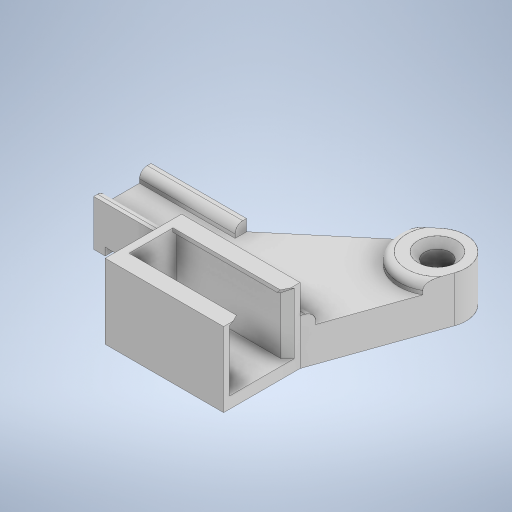
# Autodesk Inventor part: Strain Relief
Saved by Autodesk Inventor 2023.1 (Build 271208000, 208)
## iProperties
Created: 2022-11-07
Part Number: Strain Relief
Material: Generic
Document SubType Name: Modeling
Designer: nicol
Density: 1 g/cm^3
Appearance: Default
Author: nicol
Autodesk Inventor part; units mm, degrees
ref_plane "YZ Plane" through (0, 0, 0) normal (1, 0, 0) x (0, 1, 0)
ref_plane "XZ Plane" through (0, 0, 0) normal (0, 1, 0) x (-1, 0, 0)
ref_plane "XY Plane" through (0, 0, 0) normal (0, 0, 1) x (1, 0, 0)
sketch "Sketch1" plane through (0, 0, 0) normal (0, 1, 0) x (-1, 0, 0)
  circle A0 centre (-32.475, -32.475) radius 3.3
  circle A1 centre (-32.475, -32.475) radius 7.5
  line L0 (25, 0) -> (0, 0)
  line L1 (0, 0) -> (0, -15)
  line L2 (0, -15) -> (25, -15)
  line L3 (25, -15) -> (25, 0)
  line L4 (0, 20) -> (-29, 20)
  line L5 (-29, 20) -> (-29, 0)
  line L6 (-29, 0) -> (0, 0)
  line L7 (0, 0) -> (0, 20)
  line L8 (0, 0) -> (-36.8411, -26.3768)
  line L9 (0, -15) -> (-27.6522, -38.2187)
  line L10 (-29, 0) -> (-39.5499, -29.9858)
  line L11 (0, 0) -> (-55.6524, 0) construction
  line L12 (-55.6524, 0) -> (-55.6524, -63.0935) construction
  line L13 (-55.6524, -63.0935) -> (0, -63.0935) construction
  line L14 (0, -63.0935) -> (0, 0) construction
  dimension "d0" = 6.6
  dimension "d1" = 32.475
  dimension "d2" = 32.475
  dimension "d3" = 15
  dimension "d4" = 25
  dimension "d6" = 15
  dimension "d7" = 29
  dimension "d8" = 20
  constraints: 30 end point, 6 parallel, 3 horizontal, 3 perpendicular, 3 point on circle, 3 tangent, 2 centre point, 2 coincident, 2 collinear
  measures "d0" diameter of A0
  measures "d1" distance from line of A0.centre L14
  measures "d2" distance from line of L11 A0.centre
  measures "d3" distance of L2.end L0.start
  measures "d4" distance of L1.end L2.end
  measures "d6" diameter of A1
  measures "d7" distance of L4.start L4.end
  measures "d8" distance of L6.end L4.start
extrude "Extrusion1" add sketch "Sketch1" along normal blind 12
sketch "Sketch2" plane through (0, 12, 0) normal (0, 1, 0) x (1, 0, 0)
  circle A0 centre (32.475, 32.475) radius 3.3 projected
  circle A1 centre (32.475, 32.475) radius 10
  line L0 (-25, 15) -> (-25, 0) projected
  line L1 (-25, 0) -> (0, 0) projected
  line L2 (0, 0) -> (0, -20) projected
  line L3 (0, -20) -> (29, -20) projected
  line L4 (29, -20) -> (29, 0) projected
  line L5 (29, 0) -> (39.5499, 29.9858) projected
  arc A2 (39.5499, 29.9858) -> (27.6522, 38.2187) centre (32.475, 32.475) ccw projected
  line L6 (27.6522, 38.2187) -> (0, 15) projected
  line L7 (0, 15) -> (-25, 15) projected
  circle A3 centre (32.475, 32.475) radius 3.3 projected
  line L8 (-25, 15) -> (-25, 0) projected
  line L9 (-25, 12) -> (0, 12)
  line L10 (0, 12) -> (0, 3)
  line L11 (0, 3) -> (-25, 3)
  line L12 (-25, 3) -> (-25, 12)
  line L13 (27.6522, 38.2187) -> (0, 15) projected
  line L14 (0, 15) -> (0, 0)
  line L15 (29, 0) -> (39.5499, 29.9858) projected
  line L16 (0, 0) -> (30.0555, 0)
  line L17 (30.0555, 0) -> (30.0555, 3)
  line L18 (30.0555, 3) -> (0, 3)
  line L19 (0, 3) -> (0, 0)
  point P0 (37.3547, 23.7464)
  point P1 (22.5867, 33.9654)
  point P2 (-25, 7.5)
  point P3 (-25, 3)
  point P4 (29, 0)
  point P5 (29, 0)
  dimension "d11" = 20
  dimension "d14" = 9
  constraints: 18 end point, 4 parallel, 3 point on line, 2 horizontal, 2 midpoint, 2 perpendicular, 1 centre point, 1 coincident, 1 collinear, 1 vertical
  measures "d11" diameter of A1
  measures "d14" distance of L9.end L10.end
extrude "Extrusion2" cut sketch "Sketch2" against normal blind 3 contours A1 L5 L18 L10 L14 L6 | L17 L16 L5 | L10 L11 L0 L9
extrude "Extrusion7" cut sketch "Sketch2" against normal blind 9 contours L4 L3 L2 L16
sketch "Sketch3" plane through (0, 3, 0) normal (0, 1, 0) x (1, 0, 0)
  line L0 (0, -16.75) -> (29, -16.75)
  line L1 (29, -16.75) -> (29, -3.25)
  line L2 (29, -3.25) -> (0, -3.25)
  line L3 (0, -3.25) -> (0, -16.75)
  line L4 (37.3547, 23.7464) -> (30.0555, 3) projected
  arc A0 (22.5867, 33.9654) -> (37.3547, 23.7464) centre (32.475, 32.475) ccw projected
  line L5 (0, 15) -> (22.5867, 33.9654) projected
  line L6 (0, 12) -> (0, 15) projected
  line L7 (-25, 12) -> (0, 12) projected
  line L8 (-25, 3) -> (-25, 12) projected
  line L9 (30.0555, 3) -> (-25, 3) projected
  line L10 (0, 0) -> (29, 0)
  line L11 (29, 0) -> (29, -20) projected
  line L12 (0, 0) -> (29, 0) projected
  line L13 (0, -20) -> (0, 0) projected
  line L14 (29, -20) -> (0, -20) projected
  point P0 (29, -10)
  point P1 (0, -10)
  point P2 (0, -3.25)
  dimension "d15" = 13.5
  constraints: 10 end point, 3 midpoint, 2 horizontal, 2 parallel, 1 perpendicular
  measures "d15" distance of L1.end L0.end
extrude "Extrusion3" add sketch "Sketch3" along normal blind 16.5 contours L0 L11 L14 L13 | L13 L10 L11 L2
sketch "Sketch4" plane through (29, 0, 20) normal (1, 0, 0) x (0, 0, -1)
  line L0 (3.25, 19.5) -> (4.25, 19.5)
  line L1 (16.75, 19.5) -> (15.75, 19.5)
  line L2 (0, 0) -> (0, 19.5) projected
  line L3 (0, 0) -> (20, 0) projected
  line L4 (20, 0) -> (20, 12) projected
  line L5 (4.25, 19.5) -> (4.25, 18.5)
  line L6 (4.25, 18.5) -> (3.25, 17.9226)
  line L7 (15.75, 19.5) -> (15.75, 18.5)
  line L8 (15.75, 18.5) -> (16.75, 17.9226)
  line L9 (16.75, 3) -> (3.25, 3) projected
  line L10 (3.25, 3) -> (3.25, 19.5) projected
  line L11 (0, 19.5) -> (3.25, 19.5) projected
  line L12 (20, 12) -> (20, 19.5) projected
  line L13 (16.75, 19.5) -> (20, 19.5) projected
  line L14 (16.75, 3) -> (16.75, 19.5) projected
  line L15 (16.75, 3) -> (16.75, 19.5) projected
  point P0 (3.25, 23.5)
  point P1 (16.75, 23.5)
  dimension "d18" = 1
  dimension "d20" = 1
  dimension "d27" = 1
  dimension "d28" = 120
  dimension "d29" = 1
  dimension "d30" = 120
  constraints: 12 end point, 2 horizontal, 2 vertical, 1 point on line
  measures "d18" distance of L1.start L1.end
  measures "d20" distance of L0.start L0.end
  measures "d27" distance of L1.end L7.end
  measures "d28" angle of L7 L8
  measures "d29" distance of L0.end L5.end
  measures "d30" angle of L6 L5
extrude "Extrusion4" add sketch "Sketch4" against normal up to surface (29 mm away) contours L0 L5 L6 L10 | L8 L7 L1 L14
sketch "Sketch5" plane through (0, 0, 0) normal (-1, 0, 0) x (0, 0, 1)
  line L0 (0, 0) -> (20, 0) projected
  line L1 (0, 19.5) -> (4.25, 19.5) projected
  line L2 (3.25, 19.5) -> (16.75, 19.5)
  line L3 (0, 0) -> (0, 12) projected
  line L4 (16.75, 3) -> (3.25, 3) projected
  line L5 (3.25, 3) -> (3.25, 17.9226) projected
  line L6 (0, 12) -> (0, 19.5) projected
  line L7 (20, 0) -> (20, 19.5) projected
  line L8 (15.75, 19.5) -> (20, 19.5) projected
  line L9 (16.75, 3) -> (16.75, 17.9226) projected
  line L10 (4.25, 18.5) -> (3.25, 17.9226) projected
  line L11 (4.25, 19.5) -> (4.25, 18.5) projected
  line L12 (15.75, 18.5) -> (15.75, 19.5) projected
  line L13 (16.75, 17.9226) -> (15.75, 18.5) projected
  constraints: 2 end point
extrude "Extrusion5" add sketch "Sketch5" along normal blind 2
sketch "Sketch6" plane through (0, 0, 0) normal (0, -1, 0) x (1, 0, 0)
  line L0 (0, -15) -> (-25, -15) projected
  line L1 (-25, 0) -> (-2, 0) projected
  line L2 (-22, -15) -> (-19, -15)
  line L3 (-19, -15) -> (-19, 0)
  line L4 (-19, 0) -> (-22, 0)
  line L5 (-22, 0) -> (-22, -15)
  line L6 (-6, -15) -> (-3, -15)
  line L7 (-3, -15) -> (-3, 0)
  line L8 (-3, 0) -> (-6, 0)
  line L9 (-6, 0) -> (-6, -15)
  line L10 (-25, -15) -> (-25, 0) projected
  point P0 (0, 0)
  point P1 (-3, 0)
  point P2 (-22, 0)
  point P3 (-19, -15)
  dimension "d31" = 3
  dimension "d32" = 3
  dimension "d33" = 3
  dimension "d34" = 3
  constraints: 16 end point, 4 parallel, 4 point on line, 2 horizontal, 2 perpendicular
  measures "d31" distance between parallel lines of L5 L3
  measures "d32" distance between parallel lines of L9 L7
  measures "d33" distance between parallel lines of L10 L5
  measures "d34" distance from line of L0.start L7
extrude "Extrusion6" cut sketch "Sketch6" against normal blind 2 contours L0 L9 L1 L7 | L0 L5 L1 L3
chamfer "Chamfer1" distance 1.75 angle 45 8 edges at (29, 18.2113, 3.75) (29, 18.2113, 16.25) (29, 19, 4.25) (29, 19, 15.75) (29, 10.4613, 3.25) (29, 10.4613, 16.75) (35.775, 12, -32.475) (35.775, 0, -32.475)
fillet "Fillet1" radius 2 3 edges at (2.5277, 12, -3) (-12.5, 12, -12) (26.7848, 12, -24.2518)
equation "\"d2\" = d1"
body "Solid1"
